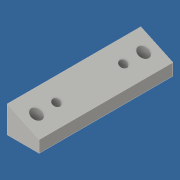
# Autodesk Inventor part: Mount
Saved by Autodesk Inventor 2016 (Build 200138000, 138)
## iProperties
Created: 2017-06-20
Part Number: Mount
Material: Generisch
Document SubType Name: Modeling
Designer: 4ndreas
Density: 1 g/cm^3
Appearance: Vorgabe
Author: 4ndreas
Autodesk Inventor part; units mm, degrees
ref_plane "YZ Plane" through (0, 0, 0) normal (1, 0, 0) x (0, 1, 0)
ref_plane "XZ Plane" through (0, 0, 0) normal (0, 1, 0) x (-1, 0, 0)
sketch "Skizze1" plane through (0, 0, 0) normal (0, 0, 1) x (1, 0, 0)
  line L0 (-6, -25) -> (6, -25)
  line L1 (6, -25) -> (6, 25)
  line L2 (6, 25) -> (-6, 25)
  line L3 (-6, 25) -> (-6, -25)
  line L4 (-6, -25) -> (6, 25) construction
  line L5 (6, -25) -> (-6, 25) construction
  line L6 (0, 20) -> (0, -20)
  point P0 (0, 0)
  point P1 (0, 0)
  dimension "d0" = 40
  dimension "d1" = 12
  dimension "d2" = 50
  constraints: 14 end point, 4 midpoint, 2 parallel, 1 horizontal, 1 perpendicular, 1 vertical
  measures "d0" distance of L6.start L6.end
  measures "d1" distance between parallel lines of L3 L1
  measures "d2" distance between parallel lines of L0 L2
extrude "Extrusion1" add sketch "Skizze1" along normal blind 10
sketch "Skizze3" plane through (0, 0, 10) normal (0, 0, 1) x (1, 0, 0)
  line L0 (-6, -25) -> (6, -25) projected
  line L1 (6, -25) -> (6, 25) projected
  line L2 (6, 25) -> (-6, 25) projected
  line L3 (-6, 25) -> (-6, -25) projected
  point P0 (0, 0)
  point P1 (0, -20)
  point P2 (0, 20)
sketch "Skizze2" plane through (-6, -25, 0) normal (0, -1, 0) x (1, 0, 0)
  line L0 (0, 0) -> (12, 0) projected
  line L1 (12, 0) -> (12, 10) projected
  line L2 (0, 10) -> (12, 10) projected
  line L3 (0, 0) -> (0, 10) projected
  line L4 (0, 10) -> (12, 4.4043)
  point P0 (6, 0)
  dimension "d5" = 25
  constraints: 2 end point, 1 point on line
  measures "d5" angle of L4 L2
extrude "Extrusion2" cut sketch "Skizze2" against normal through all contours L2 L1 L4
hole "Bohrung1" at (0, 20, 10) at (0, -20, 10) direction (0, 0, -1) diameter 3 end through all counterbore diameter 4 counterbore depth 7
sketch "Skizze4" plane through (-6, -25, 10) normal (0.4226, 0, 0.9063) x (0.9063, 0, -0.4226)
  ellipse E0 centre (6.6203, 45) end of major axis (8.827, 45) minor radius 2 projected
  ellipse E1 centre (6.6203, 5) end of major axis (8.827, 5) minor radius 2 projected
  line L0 (0, 50) -> (13.2405, 50) projected
  line L1 (0, 50) -> (0, 0) projected
  line L2 (13.2405, 0) -> (0, 0) projected
  line L3 (13.2405, 50) -> (13.2405, 0) projected
  line L4 (6.6203, 12.5) -> (6.6203, 37.5)
  line L5 (0, 50) -> (0, 0) projected
  line L6 (0, 25) -> (13.2405, 25)
  line L7 (13.2405, 50) -> (13.2405, 0) projected
  point P0 (9.664, 25)
  point P1 (6.6203, 25)
  dimension "d15" = 25
  constraints: 4 end point, 4 midpoint, 1 vertical, 2 other
  measures "d15" distance of L4.start L4.end
hole "Bohrung2" at (0, -12.5, 7.2022) at (0, 12.5, 7.2022) direction (-0.4226, 0, -0.9063) diameter 3 end through all
ref_plane "Arbeitsebene1" through (-6, 25, 0) normal (0.4226, 0, 0.9063) x (0.9063, 0, -0.4226)
sketch "Skizze5" plane through (-6, 25, 0) normal (0.4226, 0, 0.9063) x (0.9063, 0, -0.4226)
  circle A0 centre (2.3941, -37.5) radius 1.5 projected
  circle A1 centre (2.3941, -12.5) radius 1.5 projected
  ellipse E0 centre (2.3941, -5) end of major axis (4.6008, -5) minor radius 2 projected
  ellipse E1 centre (2.3941, -45) end of major axis (4.6008, -45) minor radius 2 projected
  line L0 (-4.2262, 0) -> (9.0144, 0) projected
  line L1 (-4.2262, 0) -> (-4.2262, -50) projected
  line L2 (9.0144, -50) -> (-4.2262, -50) projected
  line L3 (9.0144, 0) -> (9.0144, -50) projected
  point P0 (5.4378, -25)
  constraints: 2 other
hole "Bohrung3" at (-3.8302, 12.5, -1.0118) at (-3.8302, -12.5, -1.0118) direction (0.4226, 0, 0.9063) diameter 3 end through all counterbore diameter 4 counterbore depth 5
